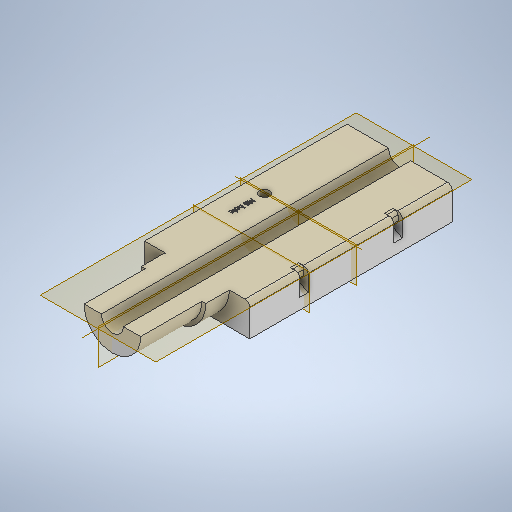
# Autodesk Inventor part: Pen_Housing_Bottom_V2
Saved by Autodesk Inventor 2025 (Build 290162000, 162)
## iProperties
Created: 2024-05-30
Part Number: Pen_Housing_Bottom_V2
Material: Generic
Document SubType Name: Modeling
Designer: mumin
Density: 1 g/cm^3
Appearance: Default
Author: mumin
Autodesk Inventor part; units mm, degrees
sketch "Sketch1" plane through (0, 0, 0) normal (1, 0, 0) x (0, 1, 0)
  line L0 (-20.5, -64.5) -> (0, -64.5)
  line L1 (0, -64.5) -> (0, 64.5)
  line L2 (0, 64.5) -> (-20.5, 64.5)
  line L3 (-20.5, 64.5) -> (-20.5, -64.5)
  line L4 (-20.5, -64.5) -> (0, 64.5) construction
  line L5 (0, -64.5) -> (-20.5, 64.5) construction
  line L6 (-24.6, 0) -> (4.1, 0) projected
  point P0 (0, 0)
  point P1 (-10.25, 0)
  dimension "d0" = 20.5
  dimension "d1" = 129
  constraints: 12 end point, 4 midpoint, 2 parallel, 1 horizontal, 1 perpendicular
  measures "d0" distance of L1.end L2.end
  measures "d1" distance of L2.end L0.start
extrude "Extrusion1" add sketch "Sketch1" along normal mid plane 67
sketch "Sketch2" plane through (-33.5, -20.5, 64.5) normal (0, 0, 1) x (1, 0, 0)
  line L0 (0, 20.5) -> (67, 20.5) projected
  arc A0 (13, 20.5) -> (54, 20.5) centre (33.5, 20.5) ccw
  line L1 (33.5, 20.5) -> (54, 20.5) construction
  line L2 (33.5, 20.5) -> (13, 20.5) construction
  point P0 (54, 20.5)
  dimension "d4" = 20.5
  dimension "d5" = 180
  constraints: 4 end point, 2 point on circle, 1 centre point, 1 coincident, 1 point on line
  measures "d4" radius of A0
  measures "d5" angle of L2 L1
extrude "Extrusion2" add sketch "Sketch2" along normal blind 15
sketch "Sketch3" plane through (-33.5, -20.5, 79.5) normal (0, 0, 1) x (1, 0, 0)
  line L0 (67, 20.5) -> (0, 20.5) projected
  arc A0 (15.5, 20.5) -> (51.5, 20.5) centre (33.5, 20.5) ccw
  line L1 (33.5, 20.5) -> (15.5, 20.5) construction
  line L2 (33.5, 20.5) -> (51.5, 20.5) construction
  dimension "d8" = 18
  dimension "d9" = 180
  constraints: 4 end point, 2 point on circle, 1 centre point, 1 coincident, 1 point on line
  measures "d8" radius of A0
  measures "d9" angle of L1 L2
extrude "Extrusion3" add sketch "Sketch3" along normal blind 39
sketch "Sketch4" plane through (33.5, 0, -64.5) normal (0, 0, -1) x (-1, 0, 0)
  line L0 (0, 0) -> (67, 0) projected
  arc A0 (26.5, 0) -> (40.5, 0) centre (33.5, 0) ccw
  line L1 (33.5, 0) -> (40.5, 0) construction
  line L2 (33.5, 0) -> (26.5, 0) construction
  point P0 (40.5, 0)
  dimension "d12" = 7
  dimension "d13" = 180
  constraints: 4 end point, 2 point on circle, 1 centre point, 1 coincident, 1 point on line
  measures "d12" radius of A0
  measures "d13" angle of L1 L2
extrude "Extrusion4" cut sketch "Sketch4" against normal through all
ref_plane "Work Plane1" through (0, 0, 30) normal (0, 0, 1) x (1, 0, 0)
sketch "Sketch5" plane through (0, 0, 30) normal (0, 0, 1) x (1, 0, 0)
  line L0 (33.5, -2) -> (33.5, -10.1)
  arc A0 (25.8, -8) -> (26.8834, -9.8375) centre (27.9, -8) ccw
  line L1 (25.8, -8) -> (25.8, -4.9024)
  arc A1 (27.8704, -6.2736) -> (25.8, -4.9024) centre (25.9, -7) ccw
  line L2 (28.8087, -6.9278) -> (29.3, -6.9278)
  line L3 (30.8, -5.4278) -> (30.8, -2)
  arc A2 (30.8, -2) -> (29.0387, -0.1051) centre (28.9, -2) ccw
  line L4 (29.0387, -0.1051) -> (27.6036, 0)
  line L5 (31.5, 0) -> (27.6036, 0)
  arc A3 (32.6591, -0.3701) -> (31.5, 0) centre (31.5, -2) ccw
  arc A4 (29.3, -6.9278) -> (30.8, -5.4278) centre (29.3, -5.4278) ccw
  line L6 (26.8834, -9.8375) -> (33.5, -13.4982)
  line L7 (33.5, -13.4982) -> (33.5, -10.1)
  arc A5 (27.8704, -6.2736) -> (28.8087, -6.9278) centre (28.8087, -5.9278) ccw
  line L8 (-53.4107, 0) -> (47.9851, 0) projected
  line L9 (33.5, -20.5) -> (33.5, 0) projected
  point P0 (0, 0)
  point P1 (33.4, 0)
  point P2 (33.5, 0)
  point P3 (33.5, -8)
  point P4 (31.4, -10.1)
  point P5 (27.9988, -6.9278)
  point P6 (30.8, -6.9278)
  point P7 (31.5, 0)
  dimension "d17" = 2
  dimension "d18" = 1.5
  dimension "d19" = 1
  constraints: 16 end point, 13 point on circle, 8 tangent, 7 point on line, 6 centre point, 1 collinear
  measures "d17" radius of A3
  measures "d18" radius of A4
  measures "d19" radius of A5
extrude "Extrusion5" cut sketch "Sketch5" along normal mid plane 5.4
mirror "Mirror1" about plane through (0, 0, 0) normal (0, 0, 1) of "Extrusion5"
fillet "Fillet1" radius 3 3 edges at (33.5, 0, 48.6) (33.5, 0, 0) (33.5, 0, -48.6)
sketch "Sketch6" plane through (-33.5, 0, 64.5) normal (0, 1, 0) x (1, 0, 0)
  line L0 (80.4, 64.5) -> (-13.4, 64.5) projected
  line L1 (0, 0) -> (0, 129) projected
  point P0 (33.5, 64.5)
  point P1 (12, 64.5)
  dimension "d30" = 12
  constraints: 1 point on line
  measures "d30" distance from line of L1 point (12, 64.5)
hole "Hole1" at (-21.5, 0, 0) direction (0, -1, 0) diameter 6.2 depth 10
sketch "Sketch7" plane through (-33.5, 0, 64.5) normal (0, 1, 0) x (1, 0, 0)
  line L0 (13.549, 57.6573) -> (13.549, 43.0546) construction
  line L1 (13.549, 43.0546) -> (10.1361, 43.0546) construction
  line L2 (10.1361, 43.0546) -> (10.1361, 57.6573) construction
  line L3 (10.1361, 57.6573) -> (13.549, 57.6573) construction
  line L4 (10.3652, 54.7353) -> (10.3652, 55.1404)
  line L5 (10.3652, 55.1404) -> (12.9908, 55.1404)
  line L6 (12.9908, 55.1404) -> (11.205, 55.9357)
  line L7 (11.205, 55.9357) -> (11.205, 56.1827)
  line L8 (11.205, 56.1827) -> (12.9908, 56.9707)
  line L9 (12.9908, 56.9707) -> (10.3652, 56.9707)
  line L10 (10.3652, 56.9707) -> (10.3652, 57.3486)
  line L11 (10.3652, 57.3486) -> (13.4132, 57.3486)
  line L12 (13.4132, 57.3486) -> (13.4132, 56.7953)
  line L13 (13.4132, 56.7953) -> (11.7163, 56.0345)
  line L14 (11.7163, 56.0345) -> (13.4132, 55.2984)
  line L15 (13.4132, 55.2984) -> (13.4132, 54.7353)
  line L16 (13.4132, 54.7353) -> (10.3652, 54.7353)
  spline S0 degree 2 poles (11.3532, 52.2776) (11.1185, 52.2776) (10.7209, 52.4332) (10.5875, 52.5641) knots 0 0 0 1 2 2 2
  spline S1 degree 2 poles (10.5875, 52.5641) (10.4467, 52.7) (10.301, 53.0409) (10.301, 53.2459) knots 0 0 0 1 2 2 2
  spline S2 degree 2 poles (10.301, 53.2459) (10.301, 53.4509) (10.4393, 53.7893) (10.5776, 53.9177) knots 0 0 0 1 2 2 2
  spline S3 degree 2 poles (10.5776, 53.9177) (10.7431, 54.0758) (11.2989, 54.2536) (11.7039, 54.2536) knots 0 0 0 1 2 2 2
  spline S4 degree 2 poles (11.7039, 54.2536) (12.1016, 54.2536) (12.7413, 54.0906) (12.9785, 53.9202) knots 0 0 0 1 2 2 2
  spline S5 degree 2 poles (12.9785, 53.9202) (13.2106, 53.7547) (13.47, 53.231) (13.47, 52.8877) knots 0 0 0 1 2 2 2
  spline S6 degree 2 poles (13.47, 52.8877) (13.47, 52.7864) (13.4502, 52.6086) (13.428, 52.5419) knots 0 0 0 1 2 2 2
  line L17 (13.428, 52.5419) -> (13.0353, 52.5419)
  line L18 (13.0353, 52.5419) -> (13.0353, 52.5592)
  spline S7 degree 2 poles (13.0353, 52.5592) (13.0649, 52.616) (13.1168, 52.8235) (13.1168, 52.9421) knots 0 0 0 1 2 2 2
  spline S8 degree 2 poles (13.1168, 52.9421) (13.1168, 53.3224) (12.603, 53.7893) (12.0991, 53.8337) knots 0 0 0 1 2 2 2
  spline S9 degree 2 poles (12.0991, 53.8337) (12.2004, 53.688) (12.3116, 53.3817) (12.3116, 53.1989) knots 0 0 0 1 2 2 2
  spline S10 degree 2 poles (12.3116, 53.1989) (12.3116, 53.0211) (12.2399, 52.7543) (12.1313, 52.6086) knots 0 0 0 1 2 2 2
  spline S11 degree 2 poles (12.1313, 52.6086) (12.0053, 52.4406) (11.615, 52.2776) (11.3532, 52.2776) knots 0 0 0 1 2 2 2
  spline S12 degree 2 poles (11.3359, 52.6926) (11.5236, 52.6926) (11.778, 52.7914) (11.867, 52.9001) knots 0 0 0 1 2 2 2
  spline S13 degree 2 poles (11.867, 52.9001) (11.9312, 52.9816) (11.9732, 53.1841) (11.9732, 53.2903) knots 0 0 0 1 2 2 2
  spline S14 degree 2 poles (11.9732, 53.2903) (11.9732, 53.4336) (11.8867, 53.7028) (11.8052, 53.8337) knots 0 0 0 1 2 2 2
  spline S15 degree 2 poles (11.8052, 53.8337) (11.7607, 53.8362) (11.6768, 53.8411) (11.6125, 53.8411) knots 0 0 0 1 2 2 2
  spline S16 degree 2 poles (11.6125, 53.8411) (11.2964, 53.8411) (10.9086, 53.7176) (10.8073, 53.6238) knots 0 0 0 1 2 2 2
  spline S17 degree 2 poles (10.8073, 53.6238) (10.711, 53.5373) (10.6344, 53.3496) (10.6344, 53.2434) knots 0 0 0 1 2 2 2
  spline S18 degree 2 poles (10.6344, 53.2434) (10.6344, 52.9964) (10.9852, 52.6926) (11.3359, 52.6926) knots 0 0 0 1 2 2 2
  line L19 (10.3652, 48.7554) -> (10.3652, 49.1407)
  line L20 (10.3652, 49.1407) -> (11.6694, 49.1407)
  spline S19 degree 2 poles (11.6694, 49.1407) (11.8274, 49.1407) (12.0991, 49.1703) (12.1807, 49.2148) knots 0 0 0 1 2 2 2
  spline S20 degree 2 poles (12.1807, 49.2148) (12.2671, 49.2617) (12.3511, 49.4297) (12.3511, 49.573) knots 0 0 0 1 2 2 2
  spline S21 degree 2 poles (12.3511, 49.573) (12.3511, 49.7162) (12.1979, 50.02) (12.0744, 50.1658) knots 0 0 0 1 2 2 2
  line L21 (12.0744, 50.1658) -> (10.3652, 50.1658)
  line L22 (10.3652, 50.1658) -> (10.3652, 50.5511)
  line L23 (10.3652, 50.5511) -> (13.549, 50.5511)
  line L24 (13.549, 50.5511) -> (13.549, 50.1658)
  line L25 (13.549, 50.1658) -> (12.398, 50.1658)
  spline S22 degree 2 poles (12.398, 50.1658) (12.5536, 49.9929) (12.7166, 49.6594) (12.7166, 49.4717) knots 0 0 0 1 2 2 2
  spline S23 degree 2 poles (12.7166, 49.4717) (12.7166, 49.1358) (12.272, 48.7554) (11.8497, 48.7554) knots 0 0 0 1 2 2 2
  line L26 (11.8497, 48.7554) -> (10.3652, 48.7554)
  spline S24 degree 2 poles (11.5088, 46.3348) (10.9308, 46.3348) (10.301, 46.8905) (10.301, 47.3549) knots 0 0 0 1 2 2 2
  spline S25 degree 2 poles (10.301, 47.3549) (10.301, 47.8316) (10.9506, 48.3775) (11.5088, 48.3775) knots 0 0 0 1 2 2 2
  spline S26 degree 2 poles (11.5088, 48.3775) (12.0818, 48.3775) (12.7166, 47.8143) (12.7166, 47.3549) knots 0 0 0 1 2 2 2
  spline S27 degree 2 poles (12.7166, 47.3549) (12.7166, 46.8905) (12.0843, 46.3348) (11.5088, 46.3348) knots 0 0 0 1 2 2 2
  spline S28 degree 2 poles (11.5088, 46.7324) (11.9534, 46.7324) (12.3857, 47.056) (12.3857, 47.3549) knots 0 0 0 1 2 2 2
  spline S29 degree 2 poles (12.3857, 47.3549) (12.3857, 47.6537) (11.9534, 47.9798) (11.5088, 47.9798) knots 0 0 0 1 2 2 2
  spline S30 degree 2 poles (11.5088, 47.9798) (11.0766, 47.9798) (10.632, 47.6537) (10.632, 47.3549) knots 0 0 0 1 2 2 2
  spline S31 degree 2 poles (10.632, 47.3549) (10.632, 47.0585) (11.0691, 46.7324) (11.5088, 46.7324) knots 0 0 0 1 2 2 2
  line L27 (10.3652, 45.5468) -> (10.3652, 45.9321)
  line L28 (10.3652, 45.9321) -> (13.549, 45.9321)
  line L29 (13.549, 45.9321) -> (13.549, 45.5468)
  line L30 (13.549, 45.5468) -> (10.3652, 45.5468)
  spline S32 degree 2 poles (10.3133, 43.9882) (10.3133, 44.5366) (10.9284, 45.1393) (11.4965, 45.1393) knots 0 0 0 1 2 2 2
  spline S33 degree 2 poles (11.4965, 45.1393) (12.0547, 45.1393) (12.7166, 44.5539) (12.7166, 44.0821) knots 0 0 0 1 2 2 2
  spline S34 degree 2 poles (12.7166, 44.0821) (12.7166, 43.8697) (12.5931, 43.5412) (12.4622, 43.4201) knots 0 0 0 1 2 2 2
  spline S35 degree 2 poles (12.4622, 43.4201) (12.3313, 43.2966) (11.9534, 43.1657) (11.6792, 43.1657) knots 0 0 0 1 2 2 2
  line L31 (11.6792, 43.1657) -> (11.4693, 43.1657)
  line L32 (11.4693, 43.1657) -> (11.4693, 44.749)
  spline S36 degree 2 poles (11.4693, 44.749) (11.0716, 44.749) (10.6492, 44.3489) (10.6492, 43.9932) knots 0 0 0 1 2 2 2
  spline S37 degree 2 poles (10.6492, 43.9932) (10.6492, 43.8672) (10.7061, 43.6227) (10.7505, 43.5239) knots 0 0 0 1 2 2 2
  spline S38 degree 2 poles (10.7505, 43.5239) (10.7999, 43.4201) (10.8864, 43.2769) (10.9259, 43.2299) knots 0 0 0 1 2 2 2
  line L33 (10.9259, 43.2299) -> (10.9259, 43.2077)
  line L34 (10.9259, 43.2077) -> (10.506, 43.2077)
  spline S39 degree 2 poles (10.506, 43.2077) (10.4788, 43.2744) (10.3998, 43.477) (10.3775, 43.556) knots 0 0 0 1 2 2 2
  spline S40 degree 2 poles (10.3775, 43.556) (10.3454, 43.6671) (10.3133, 43.8499) (10.3133, 43.9882) knots 0 0 0 1 2 2 2
  spline S41 degree 2 poles (11.7632, 43.5412) (11.9188, 43.5461) (12.1461, 43.6103) (12.2226, 43.6721) knots 0 0 0 1 2 2 2
  spline S42 degree 2 poles (12.2226, 43.6721) (12.3091, 43.7388) (12.4005, 43.9487) (12.4005, 44.1043) knots 0 0 0 1 2 2 2
  spline S43 degree 2 poles (12.4005, 44.1043) (12.4005, 44.2575) (12.3091, 44.4724) (12.2202, 44.5613) knots 0 0 0 1 2 2 2
  spline S44 degree 2 poles (12.2202, 44.5613) (12.1288, 44.6477) (11.9089, 44.7367) (11.7632, 44.749) knots 0 0 0 1 2 2 2
  line L35 (11.7632, 44.749) -> (11.7632, 43.5412)
  point P0 (33.5, 64.5)
  constraints: 2 other
emboss "Emboss1" sketch "Sketch7" operation cut depth 1 direction (0, -1, 0)
body "Solid1"
